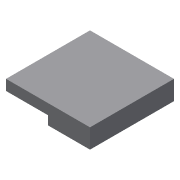
# Autodesk Inventor part: ToteBasinBracket
Saved by Autodesk Inventor 2015 (Build 190159000, 159)
## iProperties
Created: 2015-03-08
Part Number: ToteBasinBracket
Material: Generic
Document SubType Name: Modeling
Designer: Jaden
Density: 1 g/cm^3
Appearance: Default
Author: Jaden
Autodesk Inventor part; units mm, degrees
ref_plane "YZ Plane" through (0, 0, 0) normal (1, 0, 0) x (0, 1, 0)
ref_plane "XZ Plane" through (0, 0, 0) normal (0, 1, 0) x (-1, 0, 0)
ref_plane "XY Plane" through (0, 0, 0) normal (0, 0, 1) x (1, 0, 0)
sketch "Sketch1" plane through (0, 0, 0) normal (0, 0, 1) x (1, 0, 0)
  line L0 (0, 0) -> (0, 5.842)
  line L1 (0, 0) -> (5.842, 0) construction
  line L2 (0, 5.842) -> (-25.4, 5.842)
  line L3 (0, 5.842) -> (25.4, 5.842) construction
  line L4 (-25.4, 5.842) -> (-25.4, 2.667)
  line L5 (-25.4, 2.667) -> (-12.7, 2.667)
  line L6 (-25.4, 2.667) -> (-12.7, 2.667) construction
  line L7 (-12.7, 2.667) -> (-12.7, 0)
  line L8 (-12.7, 0) -> (0, 0)
  dimension "d0" = 5.842
  dimension "d1" = 90
  dimension "d2" = 25.4
  dimension "d3" = 180
  dimension "d4" = 3.175
  dimension "d5" = 12.7
  dimension "d6" = 0
  constraints: 18 end point, 5 horizontal, 3 equal length, 3 perpendicular, 1 vertical
  measures "d0" distance of L0.start L0.end
  measures "d1" angle of L1 L0
  measures "d2" distance of L0.end L2.end
  measures "d3" angle of L2 L3
  measures "d4" distance of L2.end L4.end
  measures "d5" distance of L4.end L5.end
  measures "d6" distance between parallel lines of L5 L6
extrude "Extrusion1" add sketch "Sketch1" along normal blind 25.4
body "Solid1"
